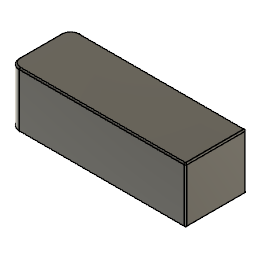
batterie (Autodesk Fusion 360 design; units mm, degrees)
Autodesk Fusion 360 part; units mm, degrees
sketch "Sketch1" plane through (0, 0, 0) normal (0, 0, 1) x (1, 0, 0)
  line L0 (69.5, -24) -> (-69.5, -24)
  line L1 (-69.5, -24) -> (-69.5, 24)
  line L2 (-69.5, 24) -> (69.5, 24)
  line L3 (69.5, 24) -> (69.5, -24)
  line L4 (69.5, -24) -> (-69.5, 24) construction
  line L5 (-69.5, -24) -> (69.5, 24) construction
  dimension "d1" = 139
  dimension "d2" = 48
  constraint horizontal L0
  constraint perpendicular L0 L1
  constraint parallel L0 L2
  constraint parallel L1 L3
  constraint coincident L4 origin
  constraint coincident L5 origin
  measures "d1" distance of L1.end L2.end
  measures "d2" distance of L0.end L1.end
extrude "Extrude1" add sketch "Sketch1" along normal blind 44
fillet "Fillet1" radius 1 2 edges at (69.5, -24, 22) (69.5, 24, 22)
fillet "Fillet2" radius 1 6 edges at (-0.5, -24, 44) (69.2071, -23.7071, 44) (69.5, 0, 44) (69.2071, 23.7071, 44) (-0.5, 24, 44) (-69.5, 0, 44)
fillet "Fillet3" radius 1 6 edges at (-0.5, 24, 0) (69.2071, 23.7071, 0) (69.5, 0, 0) (69.2071, -23.7071, 0) (-0.5, -24, 0) (-69.5, 0, 0)
fillet "Fillet4" radius 7.5 6 edges at (-69.2071, 23.7071, 0.2929) (-69.5, 24, 22) (-69.2071, 23.7071, 43.7071) (-69.2071, -23.7071, 0.2929) (-69.5, -24, 22) (-69.2071, -23.7071, 43.7071)
